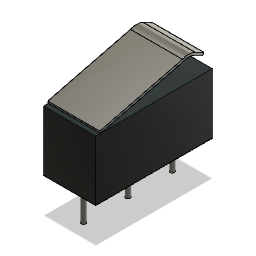
Rotary Limit Switch v1 (Autodesk Fusion 360 design; units mm, degrees)
Autodesk Fusion 360 part; units mm, degrees
sketch "Sketch1" plane through (0, 0, 0) normal (1, 0, 0) x (0, 0, -1)
  line L0 (0, 0) -> (12.8016, 0)
  line L1 (12.8016, 0) -> (12.8016, 6.604)
  line L2 (12.8016, 6.604) -> (0, 6.604)
  line L3 (0, 6.604) -> (0, 0)
  dimension "d1" = 12.8016
  dimension "d2" = 6.604
  constraint horizontal L0
  constraint vertical L1
  constraint horizontal L2
  constraint vertical L3
  constraint coincident L0.start L3.end
  measures "d1" distance of L0.start L0.end
  measures "d2" distance of L0.start L2.end
extrude "Extrude1" add sketch "Sketch1" along normal blind 5.715 makes body 1
sketch "Sketch2" plane through (0, 6.604, 0) normal (0, 1, 0) x (-1, 0, 0)
  line L0 (0, -12.8016) -> (0, 0)
  line L1 (0, 0) -> (-5.715, 0)
  line L2 (-5.715, 0) -> (-5.715, -12.8016)
  line L3 (-5.715, -12.8016) -> (0, -12.8016)
sketch "Sketch3" plane through (0, 0, 0) normal (0, -1, 0) x (1, 0, 0)
  line L0 (0, 0) -> (0, -12.8016)
  line L1 (0, -12.8016) -> (5.715, -12.8016)
  line L2 (5.715, -12.8016) -> (5.715, 0)
  line L3 (5.715, 0) -> (0, 0)
  circle A0 centre (2.8575, -1.524) radius 0.254
  line L4 (2.8575, 0) -> (2.8575, -12.8016) construction
  circle A1 centre (2.8575, -6.4008) radius 0.254
  circle A2 centre (2.8575, -11.2776) radius 0.254
  line L5 (5.715, -6.4008) -> (0, -6.4008) construction
  dimension "d5" = 0.508
  dimension "d6" = 0.508
  dimension "d7" = 0.508
  dimension "d8" = 1.524
  dimension "d9" = 1.524
  constraint midpoint L3 L4.start
  constraint midpoint L1 L4.end
  constraint coincident A0.centre L4
  constraint midpoint L2 L5.start
  constraint midpoint L0 L5.end
  constraint coincident A1.centre L5
  measures "d5" diameter of A0
  measures "d6" diameter of A1
  measures "d7" diameter of A2
  measures "d8" distance of L4.end A2.centre
  measures "d9" distance of L3 A0.centre
extrude "Extrude2" add sketch "Sketch3" along normal blind 3.81 contours A0 | A1 | A2 bodies 1
sketch "Sketch4" plane through (5.715, 0, 0) normal (1, 0, 0) x (0, 0, -1)
  line L0 (0, 6.604) -> (0, 0)
  line L1 (0, 0) -> (12.8016, 0)
  line L2 (12.8016, 0) -> (12.8016, 6.604)
  line L3 (12.8016, 6.604) -> (0, 6.604)
  line L4 (0.508, 6.604) -> (9.6237, 8.89)
  arc A0 (10.7893, 8.89) -> (9.6237, 8.89) centre (10.2065, 7.7422) ccw
  line L5 (10.7893, 8.89) -> (11.7703, 8.3919)
  line L6 (0.4462, 6.8504) -> (9.5355, 9.1297)
  arc A1 (10.9042, 9.1165) -> (9.5355, 9.1297) centre (10.2065, 7.7422) ccw
  line L7 (10.9042, 9.1165) -> (11.8853, 8.6184)
  line L8 (11.8853, 8.6184) -> (11.7703, 8.3919)
  line L9 (0.4462, 6.8504) -> (0.508, 6.604)
  point P0 (0.508, 6.604)
  dimension "d12" = 0.508
  dimension "d13" = 9.398
  dimension "d14" = 2.286
  dimension "d15" = 0.254
  constraint coincident L3 P0
  constraint coincident P0 L4.start
  constraint tangent A0 L5
  constraint perpendicular L5 L8
  constraint perpendicular L4 L9
  measures "d12" distance of L0 P0
  measures "d13" distance of P0 L4.end
  measures "d14" distance of L3 L4.end
extrude "Extrude3" add sketch "Sketch4" against normal blind 5.715 separate body contours L4 A0 L5 L6 A1 L7 L8 L9 makes body 2
